# Autodesk Inventor part: m1.5_nut
Saved by Autodesk Inventor 2021 (Build 250183000, 183)
## iProperties
Created: 2021-03-15
Part Number: m1.5_nut
Material: Stainless Steel
Document SubType Name: Modeling
Designer: Tomasz Lisowski
Density: 8 g/cm^3
Appearance: Semi-Polished
Author: Tomasz Lisowski
Autodesk Inventor part; units mm, degrees
ref_plane "YZ Plane" through (0, 0, 0) normal (1, 0, 0) x (0, 1, 0)
ref_plane "XZ Plane" through (0, 0, 0) normal (0, 1, 0) x (-1, 0, 0)
ref_plane "XY Plane" through (0, 0, 0) normal (0, 0, 1) x (1, 0, 0)
sketch "Sketch1" plane through (0, 0, 0) normal (0, 1, 0) x (-1, 0, 0)
  line L0 (-1.5, -0.866) -> (-1.5, 0.866)
  line L1 (-1.5, 0.866) -> (0, 1.7321)
  line L2 (0, 1.7321) -> (1.5, 0.866)
  line L3 (1.5, 0.866) -> (1.5, -0.866)
  line L4 (1.5, -0.866) -> (0, -1.7321)
  line L5 (0, -1.7321) -> (-1.5, -0.866)
  circle A0 centre (0, 0) radius 0.75
  dimension "d0" = 3
  dimension "d1" = 1.5
  constraints: 12 end point, 2 coincident, 1 centre point, 1 vertical alignment, 13 other
  measures "d0" distance between parallel lines of L0 L3
  measures "d1" diameter of A0
extrude "Extrusion1" add sketch "Sketch1" along normal blind 1.1
body "Solid1"
